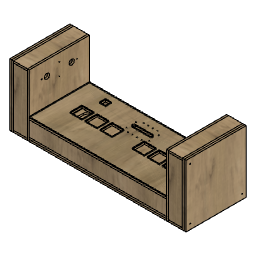
ongekicon-diy (Autodesk Fusion 360 design; units mm, degrees)
Autodesk Fusion 360 part; units mm, degrees
sketch "스케치1" plane through (0, 0, 0) normal (0, 0, 1) x (1, 0, 0)
  line L0 (289, -642.7336) -> (375, -642.7336)
  line L1 (375, -656.7336) -> (289, -656.7336)
  arc A0 (289, -642.7336) -> (289, -656.7336) centre (289, -649.7336) ccw
  arc A1 (375, -656.7336) -> (375, -642.7336) centre (375, -649.7336) ccw
  arc A2 (375, -656.7336) -> (375, -642.7336) centre (375, -649.7336) ccw
  circle A3 centre (277.0783, -626.5501) radius 2.65
  circle A4 centre (277.0783, -672.9171) radius 2.65
  circle A5 centre (386.9217, -626.4866) radius 2.65
  circle A6 centre (386.9217, -672.8535) radius 2.65
  circle A7 centre (299.0783, -611.6097) radius 2.65
  circle A8 centre (321.0783, -611.6097) radius 2.65
  circle A9 centre (343.0783, -611.6097) radius 2.65
  circle A10 centre (365.0783, -611.6097) radius 2.65
  circle A11 centre (364.9217, -687.7939) radius 2.65
  circle A12 centre (342.9217, -687.7939) radius 2.65
  circle A13 centre (320.9217, -687.7939) radius 2.65
  circle A14 centre (298.9217, -687.7939) radius 2.65
  line L2 (0, -575) -> (664, -575)
  line L3 (664, -575) -> (664, -866)
  line L4 (664, -866) -> (0, -866)
  line L5 (0, -866) -> (0, -575)
  line L6 (0, -1260) -> (664, -1260)
  line L7 (664, -1260) -> (664, -1333)
  line L8 (664, -1333) -> (0, -1333)
  line L9 (0, -1333) -> (0, -1260)
  line L10 (0, -1495) -> (0, -1422)
  line L11 (664, -1422) -> (664, -1495)
  line L12 (0, -1422) -> (664, -1422)
  line L13 (664, -1495) -> (0, -1495)
  line L14 (634, -431) -> (634, -260)
  line L15 (664, -200) -> (664, -491)
  line L16 (0, -200) -> (664, -200)
  line L17 (60, -461) -> (604, -461)
  line L18 (664, -491) -> (0, -491)
  line L19 (30, -260) -> (30, -431)
  line L20 (604, -230) -> (60, -230)
  line L21 (0, -491) -> (0, -200)
  line L22 (0, -230) -> (0, -200) construction
  arc A15 (60, -230) -> (30, -260) centre (60, -260) ccw
  arc A16 (634, -260) -> (604, -230) centre (604, -260) ccw
  arc A17 (604, -461) -> (634, -431) centre (604, -431) ccw
  arc A18 (30, -431) -> (60, -461) centre (60, -431) ccw
  circle A19 centre (644.0002, -219.9998) radius 3.25
  circle A20 centre (644.0002, -471.0002) radius 3.25
  circle A21 centre (19.9998, -219.9998) radius 3.25
  circle A22 centre (19.9998, -471.0002) radius 3.25
  line L23 (1115.742, -1032.7777) -> (1406.742, -1032.7777)
  line L24 (1406.742, -1032.7777) -> (1406.742, -1099.7777)
  line L25 (1406.742, -1099.7777) -> (1115.742, -1099.7777)
  line L26 (1115.742, -1099.7777) -> (1115.742, -1032.7777)
  line L27 (765.742, -1032.7777) -> (1056.742, -1032.7777)
  line L28 (1056.742, -1032.7777) -> (1056.742, -1099.7777)
  line L29 (1056.742, -1099.7777) -> (765.742, -1099.7777)
  line L30 (765.742, -1099.7777) -> (765.742, -1032.7777)
  line L31 (1115.742, -232.7777) -> (1406.742, -232.7777)
  line L32 (1406.742, -232.7777) -> (1406.742, -299.7777)
  line L33 (1406.742, -299.7777) -> (1115.742, -299.7777)
  line L34 (1115.742, -299.7777) -> (1115.742, -232.7777)
  line L35 (765.742, -232.7777) -> (1056.742, -232.7777)
  line L36 (1056.742, -232.7777) -> (1056.742, -299.7777)
  line L37 (1056.742, -299.7777) -> (765.742, -299.7777)
  line L38 (765.742, -299.7777) -> (765.742, -232.7777)
  line L39 (1455.3395, -732.946) -> (1522.3395, -732.946)
  line L40 (1522.3395, -732.946) -> (1522.3395, -1014.946)
  line L41 (1522.3395, -1014.946) -> (1455.3395, -1014.946)
  line L42 (1455.3395, -1014.946) -> (1455.3395, -732.946)
  line L43 (1622.3395, -1014.946) -> (1555.3395, -1014.946)
  line L44 (1555.3395, -1014.946) -> (1555.3395, -732.946)
  line L45 (1555.3395, -732.946) -> (1622.3395, -732.946)
  line L46 (1622.3395, -732.946) -> (1622.3395, -1014.946)
  line L47 (1555.3395, -664.946) -> (1555.3395, -382.946)
  line L48 (1555.3395, -382.946) -> (1622.3395, -382.946)
  line L49 (1622.3395, -382.946) -> (1622.3395, -664.946)
  line L50 (1622.3395, -664.946) -> (1555.3395, -664.946)
  line L51 (1455.3395, -664.946) -> (1455.3395, -382.946)
  line L52 (1455.3395, -382.946) -> (1522.3395, -382.946)
  line L53 (1522.3395, -664.946) -> (1455.3395, -664.946)
  line L54 (1522.3395, -382.946) -> (1522.3395, -664.946)
  line L55 (774.742, -665.946) -> (765.742, -665.946)
  line L56 (1047.742, -665.946) -> (774.742, -665.946)
  line L57 (1047.742, -665.946) -> (1056.742, -665.946)
  line L58 (1056.742, -365.946) -> (1056.742, -665.946)
  line L59 (1056.742, -365.946) -> (765.742, -365.946)
  line L60 (765.742, -365.946) -> (765.742, -665.946)
  arc A23 (1710.7461, -923.4722) -> (1740.7461, -953.4722) centre (1740.7461, -923.4722) ccw
  line L61 (1920.7461, -713.4722) -> (1740.7461, -713.4722)
  arc A24 (1740.7461, -713.4722) -> (1710.7461, -743.4722) centre (1740.7461, -743.4722) ccw
  line L62 (1710.7461, -743.4722) -> (1710.7461, -923.4722)
  circle A25 centre (1705.2461, -958.9722) radius 3.25
  circle A26 centre (1705.2461, -707.9722) radius 3.25
  line L63 (1685.2461, -683.4722) -> (1685.2461, -983.4722)
  line L64 (1976.2461, -683.4722) -> (1976.2461, -983.4722)
  line L65 (1950.7461, -923.4722) -> (1950.7461, -743.4722)
  line L66 (1740.7461, -953.4722) -> (1920.7461, -953.4722)
  arc A27 (1920.7461, -953.4722) -> (1950.7461, -923.4722) centre (1920.7461, -923.4722) ccw
  arc A28 (1950.7461, -743.4722) -> (1920.7461, -713.4722) centre (1920.7461, -743.4722) ccw
  circle A29 centre (1956.2461, -707.9722) radius 3.25
  circle A30 centre (1956.2461, -958.9722) radius 3.25
  line L67 (1976.2461, -683.4722) -> (1685.2461, -683.4722)
  line L68 (1976.2461, -983.4722) -> (1685.2461, -983.4722)
  line L69 (1976.2461, -633.4722) -> (1685.2461, -633.4722)
  line L70 (1976.2461, -333.4722) -> (1976.2461, -633.4722)
  line L71 (1710.7461, -393.4722) -> (1710.7461, -573.4722)
  line L72 (1685.2461, -333.4722) -> (1685.2461, -633.4722)
  arc A31 (1950.7461, -393.4722) -> (1920.7461, -363.4722) centre (1920.7461, -393.4722) ccw
  circle A32 centre (1956.2461, -608.9722) radius 3.25
  circle A33 centre (1705.2461, -357.9722) radius 3.25
  circle A34 centre (1956.2461, -357.9722) radius 3.25
  line L73 (1740.7461, -603.4722) -> (1920.7461, -603.4722)
  line L74 (1950.7461, -573.4722) -> (1950.7461, -393.4722)
  arc A35 (1920.7461, -603.4722) -> (1950.7461, -573.4722) centre (1920.7461, -573.4722) ccw
  line L75 (1920.7461, -363.4722) -> (1740.7461, -363.4722)
  circle A36 centre (1705.2461, -608.9722) radius 3.25
  arc A37 (1710.7461, -573.4722) -> (1740.7461, -603.4722) centre (1740.7461, -573.4722) ccw
  arc A38 (1740.7461, -363.4722) -> (1710.7461, -393.4722) centre (1740.7461, -393.4722) ccw
  line L76 (1976.2461, -333.4722) -> (1685.2461, -333.4722)
  line L77 (765.742, -704.946) -> (765.742, -1004.946)
  circle A39 centre (851.242, -774.446) radius 12.5
  line L78 (1056.742, -704.946) -> (765.742, -704.946)
  line L79 (1056.742, -1004.946) -> (765.742, -1004.946)
  circle A40 centre (971.242, -774.446) radius 12.5
  line L80 (765.742, -909.446) -> (765.742, -1004.946)
  circle A41 centre (996.242, -774.446) radius 2.2361
  circle A42 centre (826.242, -774.446) radius 2.2592
  circle A43 centre (911.242, -804.446) radius 2.2361
  line L81 (1056.742, -704.946) -> (1056.742, -1004.946)
  circle A44 centre (911.242, -744.446) radius 2.2361
  circle A45 centre (785.742, -641.446) radius 2.5
  circle A46 centre (1036.742, -641.446) radius 2.5
  circle A47 centre (1036.742, -390.446) radius 2.5
  circle A48 centre (1135.742, -390.446) radius 2.5
  line L82 (1115.742, -365.946) -> (1115.742, -665.946)
  circle A49 centre (1135.742, -641.446) radius 2.5
  line L83 (1397.742, -665.946) -> (1406.742, -665.946)
  line L84 (1397.742, -665.946) -> (1124.742, -665.946)
  line L85 (1406.742, -365.946) -> (1115.742, -365.946)
  line L86 (1406.742, -365.946) -> (1406.742, -665.946)
  line L87 (1124.742, -665.946) -> (1115.742, -665.946)
  circle A50 centre (1386.742, -641.446) radius 2.5
  circle A51 centre (1386.742, -390.446) radius 2.5
  circle A52 centre (456.3298, -1576.2079) radius 4
  circle A53 centre (547.3298, -1605.2079) radius 4
  circle A54 centre (592.8298, -1590.7079) radius 4
  circle A55 centre (547.3298, -1576.2079) radius 4
  circle A56 centre (410.8298, -1590.7079) radius 4
  circle A57 centre (501.8298, -1590.7079) radius 4
  circle A58 centre (456.3298, -1605.2079) radius 4
  line L88 (521.8298, -1571.2079) -> (481.2298, -1571.2079)
  line L89 (479.3298, -1573.1079) -> (479.3298, -1578.7079)
  line L90 (481.8298, -1581.2079) -> (521.8298, -1581.2079)
  line L91 (524.3298, -1578.7079) -> (524.3298, -1573.7079)
  arc A59 (524.3298, -1573.7079) -> (521.8298, -1571.2079) centre (521.8298, -1573.7079) ccw
  arc A60 (521.8298, -1581.2079) -> (524.3298, -1578.7079) centre (521.8298, -1578.7079) ccw
  arc A61 (479.3298, -1578.7079) -> (481.8298, -1581.2079) centre (481.8298, -1578.7079) ccw
  arc A62 (481.2298, -1571.2079) -> (479.3298, -1573.1079) centre (481.2298, -1573.1079) ccw
  line L92 (365.3298, -1554.2079) -> (638.3298, -1554.2079)
  line L93 (638.3298, -1554.2079) -> (638.3298, -1627.2079)
  line L94 (638.3298, -1627.2079) -> (365.3298, -1627.2079)
  line L95 (365.3298, -1627.2079) -> (365.3298, -1554.2079)
  arc A63 (933.742, -933.446) -> (931.242, -930.946) centre (931.242, -933.446) ccw
  line L96 (933.742, -938.446) -> (933.742, -933.446)
  line L97 (931.242, -930.946) -> (890.642, -930.946)
  arc A64 (931.242, -940.946) -> (933.742, -938.446) centre (931.242, -938.446) ccw
  arc A65 (888.742, -938.446) -> (891.242, -940.946) centre (891.242, -938.446) ccw
  circle A66 centre (865.742, -964.946) radius 4
  circle A67 centre (911.242, -950.446) radius 4
  line L98 (891.242, -940.946) -> (931.242, -940.946)
  arc A68 (890.642, -930.946) -> (888.742, -932.846) centre (890.642, -932.846) ccw
  circle A69 centre (865.742, -935.946) radius 4
  line L99 (888.742, -932.846) -> (888.742, -938.446)
  circle A70 centre (820.242, -950.446) radius 4
  circle A71 centre (1002.242, -950.446) radius 4
  circle A72 centre (956.742, -964.946) radius 4
  circle A73 centre (956.742, -935.946) radius 4
  circle A74 centre (1352.242, -950.446) radius 4
  circle A75 centre (1306.742, -935.946) radius 4
  arc A76 (1281.242, -940.946) -> (1283.742, -938.446) centre (1281.242, -938.446) ccw
  arc A77 (1283.742, -933.446) -> (1281.242, -930.946) centre (1281.242, -933.446) ccw
  line L100 (1281.242, -930.946) -> (1240.642, -930.946)
  circle A78 centre (1261.242, -950.446) radius 4
  circle A79 centre (1306.742, -964.946) radius 4
  line L101 (1406.742, -704.946) -> (1406.742, -1004.946)
  arc A80 (1238.742, -938.446) -> (1241.242, -940.946) centre (1241.242, -938.446) ccw
  circle A81 centre (1170.242, -950.446) radius 4
  line L102 (1283.742, -938.446) -> (1283.742, -933.446)
  circle A82 centre (1261.242, -744.446) radius 2.2361
  circle A83 centre (1215.742, -935.946) radius 4
  arc A84 (1240.642, -930.946) -> (1238.742, -932.846) centre (1240.642, -932.846) ccw
  line L103 (1238.742, -932.846) -> (1238.742, -938.446)
  circle A85 centre (1215.742, -964.946) radius 4
  circle A86 centre (1261.242, -804.446) radius 2.2361
  circle A87 centre (1176.242, -774.446) radius 2.2592
  line L104 (1241.242, -940.946) -> (1281.242, -940.946)
  circle A88 centre (1201.242, -774.446) radius 12.5
  line L105 (1406.742, -1004.946) -> (1115.742, -1004.946)
  line L106 (1115.742, -909.446) -> (1115.742, -1004.946)
  line L107 (1115.742, -704.946) -> (1115.742, -1004.946)
  line L108 (1406.742, -704.946) -> (1115.742, -704.946)
  circle A89 centre (1346.242, -774.446) radius 2.2361
  circle A90 centre (1321.242, -774.446) radius 12.5
  line L109 (121.8298, -1581.2079) -> (161.8298, -1581.2079)
  line L110 (161.8298, -1571.2079) -> (121.2298, -1571.2079)
  line L111 (119.3298, -1573.1079) -> (119.3298, -1578.7079)
  line L112 (278.3298, -1554.2079) -> (278.3298, -1627.2079)
  arc A91 (161.8298, -1581.2079) -> (164.3298, -1578.7079) centre (161.8298, -1578.7079) ccw
  arc A92 (119.3298, -1578.7079) -> (121.8298, -1581.2079) centre (121.8298, -1578.7079) ccw
  circle A93 centre (187.3298, -1576.2079) radius 4
  arc A94 (121.2298, -1571.2079) -> (119.3298, -1573.1079) centre (121.2298, -1573.1079) ccw
  line L113 (164.3298, -1578.7079) -> (164.3298, -1573.7079)
  circle A95 centre (187.3298, -1605.2079) radius 4
  circle A96 centre (141.8298, -1590.7079) radius 4
  arc A97 (164.3298, -1573.7079) -> (161.8298, -1571.2079) centre (161.8298, -1573.7079) ccw
  line L114 (278.3298, -1627.2079) -> (5.3298, -1627.2079)
  circle A98 centre (96.3298, -1576.2079) radius 4
  circle A99 centre (232.8298, -1590.7079) radius 4
  line L115 (5.3298, -1627.2079) -> (5.3298, -1554.2079)
  circle A100 centre (50.8298, -1590.7079) radius 4
  circle A101 centre (96.3298, -1605.2079) radius 4
  line L116 (5.3298, -1554.2079) -> (278.3298, -1554.2079)
  line L117 (138.1898, -635.6975) -> (109.1898, -635.6975)
  line L118 (109.1898, -635.6975) -> (109.1898, -606.6975)
  line L119 (109.1898, -606.6975) -> (138.1898, -606.6975)
  line L120 (138.1898, -606.6975) -> (138.1898, -635.6975)
  line L121 (525.8102, -635.6975) -> (554.8102, -635.6975)
  line L122 (554.8102, -635.6975) -> (554.8102, -606.6975)
  line L123 (554.8102, -606.6975) -> (525.8102, -606.6975)
  line L124 (525.8102, -606.6975) -> (525.8102, -635.6975)
  line L125 (554.8102, -985.6975) -> (554.8102, -956.6975)
  line L126 (109.1898, -985.6975) -> (109.1898, -956.6975)
  line L127 (138.1898, -956.6975) -> (138.1898, -985.6975)
  line L128 (525.8102, -956.6975) -> (525.8102, -985.6975)
  line L129 (525.8102, -985.6975) -> (554.8102, -985.6975)
  line L130 (664, -925) -> (664, -1216)
  line L131 (0, -1216) -> (0, -925)
  line L132 (109.1898, -956.6975) -> (138.1898, -956.6975)
  arc A102 (289, -992.7336) -> (289, -1006.7336) centre (289, -999.7336) ccw
  arc A103 (375, -1006.7336) -> (375, -992.7336) centre (375, -999.7336) ccw
  arc A104 (375, -1006.7336) -> (375, -992.7336) centre (375, -999.7336) ccw
  line L133 (138.1898, -985.6975) -> (109.1898, -985.6975)
  line L134 (375, -1006.7336) -> (289, -1006.7336)
  line L135 (664, -1216) -> (0, -1216)
  line L136 (0, -925) -> (664, -925)
  line L137 (289, -992.7336) -> (375, -992.7336)
  line L138 (554.8102, -956.6975) -> (525.8102, -956.6975)
  circle A105 centre (644, -130) radius 2.5
  circle A106 centre (644, 121) radius 2.5
  line L139 (664, 141) -> (664, -150)
  line L140 (0, 141) -> (664, 141)
  line L141 (664, -150) -> (0, -150)
  line L142 (0, -150) -> (0, 141)
  circle A107 centre (20, -130) radius 2.5
  circle A108 centre (20, 121) radius 2.5
  line L143 (180.5, -1312) -> (151.5, -1312)
  line L144 (151.5, -1312) -> (151.5, -1283)
  line L145 (151.5, -1283) -> (180.5, -1283)
  line L146 (180.5, -1283) -> (180.5, -1312)
  line L147 (318.75, -1303.75) -> (306.25, -1303.75)
  line L148 (306.25, -1303.75) -> (306.25, -1291.25)
  line L149 (306.25, -1291.25) -> (318.75, -1291.25)
  line L150 (318.75, -1291.25) -> (318.75, -1303.75)
  line L151 (483.5, -1312) -> (512.5, -1312)
  line L152 (512.5, -1312) -> (512.5, -1283)
  line L153 (483.5, -1283) -> (483.5, -1312)
  line L154 (512.5, -1283) -> (483.5, -1283)
  line L155 (357.75, -1303.75) -> (357.75, -1291.25)
  line L156 (357.75, -1291.25) -> (345.25, -1291.25)
  line L157 (345.25, -1303.75) -> (357.75, -1303.75)
  line L158 (345.25, -1291.25) -> (345.25, -1303.75)
  line L159 (136.915, -748.0793) -> (78.915, -748.0793)
  line L160 (78.915, -748.0793) -> (78.915, -690.0793)
  line L161 (78.915, -690.0793) -> (136.915, -690.0793)
  line L162 (136.915, -690.0793) -> (136.915, -748.0793)
  line L163 (209.8081, -748.0793) -> (151.8081, -748.0793)
  line L164 (151.8081, -748.0793) -> (151.8081, -690.0793)
  line L165 (151.8081, -690.0793) -> (209.8081, -690.0793)
  line L166 (209.8081, -690.0793) -> (209.8081, -748.0793)
  line L167 (282.7013, -748.0793) -> (224.7013, -748.0793)
  line L168 (224.7013, -748.0793) -> (224.7013, -690.0793)
  line L169 (224.7013, -690.0793) -> (282.7013, -690.0793)
  line L170 (282.7013, -690.0793) -> (282.7013, -748.0793)
  line L171 (512.1919, -690.0793) -> (454.1919, -690.0793)
  line L172 (527.085, -748.0793) -> (585.085, -748.0793)
  line L173 (454.1919, -748.0793) -> (512.1919, -748.0793)
  line L174 (585.085, -748.0793) -> (585.085, -690.0793)
  line L175 (381.2987, -690.0793) -> (381.2987, -748.0793)
  line L176 (381.2987, -748.0793) -> (439.2987, -748.0793)
  line L177 (454.1919, -690.0793) -> (454.1919, -748.0793)
  line L178 (585.085, -690.0793) -> (527.085, -690.0793)
  line L179 (439.2987, -690.0793) -> (381.2987, -690.0793)
  line L180 (527.085, -690.0793) -> (527.085, -748.0793)
  line L181 (512.1919, -748.0793) -> (512.1919, -690.0793)
  line L182 (439.2987, -748.0793) -> (439.2987, -690.0793)
  line L183 (152.5581, -1098.8293) -> (152.5581, -1040.8293)
  line L184 (79.665, -1098.8293) -> (79.665, -1040.8293)
  line L185 (79.665, -1040.8293) -> (137.665, -1040.8293)
  line L186 (152.5581, -1040.8293) -> (210.5581, -1040.8293)
  line L187 (137.665, -1040.8293) -> (137.665, -1098.8293)
  line L188 (210.5581, -1098.8293) -> (152.5581, -1098.8293)
  line L189 (137.665, -1098.8293) -> (79.665, -1098.8293)
  line L190 (210.5581, -1040.8293) -> (210.5581, -1098.8293)
  line L191 (225.4513, -1098.8293) -> (225.4513, -1040.8293)
  line L192 (283.4513, -1098.8293) -> (225.4513, -1098.8293)
  line L193 (225.4513, -1040.8293) -> (283.4513, -1040.8293)
  line L194 (283.4513, -1040.8293) -> (283.4513, -1098.8293)
  line L195 (526.335, -1098.8293) -> (584.335, -1098.8293)
  line L196 (526.335, -1040.8293) -> (526.335, -1098.8293)
  line L197 (380.5487, -1040.8293) -> (380.5487, -1098.8293)
  line L198 (380.5487, -1098.8293) -> (438.5487, -1098.8293)
  line L199 (453.4419, -1040.8293) -> (453.4419, -1098.8293)
  line L200 (438.5487, -1098.8293) -> (438.5487, -1040.8293)
  line L201 (438.5487, -1040.8293) -> (380.5487, -1040.8293)
  line L202 (511.4419, -1098.8293) -> (511.4419, -1040.8293)
  line L203 (453.4419, -1098.8293) -> (511.4419, -1098.8293)
  line L204 (584.335, -1098.8293) -> (584.335, -1040.8293)
  line L205 (511.4419, -1040.8293) -> (453.4419, -1040.8293)
  line L206 (584.335, -1040.8293) -> (526.335, -1040.8293)
  circle A109 centre (785.742, -390.446) radius 2.6
  line L207 (-100, 300) -> (2100, 300) construction
  line L208 (2100, 300) -> (2100, -1700) construction
  line L209 (2100, -1700) -> (-100, -1700) construction
  line L210 (-100, -1700) -> (-100, 300) construction
  line L211 (725, -150) -> (2000, -150) construction
  line L212 (2000, -150) -> (2000, -1125) construction
  line L213 (2000, -1125) -> (725, -1125) construction
  line L214 (725, -1125) -> (725, -150) construction
  line L215 (668.8847, -1871.4967) -> (1168.8847, -1871.4967) construction
  line L216 (1168.8847, -1871.4967) -> (1168.8847, -1771.4967) construction
  line L217 (1168.8847, -1771.4967) -> (668.8847, -1771.4967) construction
  line L218 (668.8847, -1771.4967) -> (668.8847, -1871.4967) construction
  line L219 (150.0308, -1682.8385) -> (548.5377, -1682.465) construction
  line L220 (548.5377, -1682.465) -> (548.5069, -1649.6265) construction
  line L221 (548.5069, -1649.6265) -> (150, -1650) construction
  line L222 (150, -1650) -> (150.0308, -1682.8385) construction
  line L223 (918.4716, -1223.3511) -> (1893.2087, -1220.0773) construction
  line L224 (1893.2087, -1220.0773) -> (1892.9571, -1145.174) construction
  line L225 (1892.9571, -1145.174) -> (918.22, -1148.4477) construction
  line L226 (918.22, -1148.4477) -> (918.4716, -1223.3511) construction
  point P0 (0, -350)
  point P1 (1830.7461, -483.4722)
  point P2 (911.242, -951.946)
  point P3 (911.242, -951.946)
  point P4 (166, -1297.5)
  point P5 (166, -1297.5)
  point P6 (501.8298, -1590.7079)
  point P7 (501.8298, -1576.2079)
  point P8 (911.242, -935.946)
  point P9 (911.242, -950.446)
  point P10 (1261.242, -951.946)
  point P11 (1261.242, -935.946)
  point P12 (1261.242, -950.446)
  point P13 (1261.242, -951.946)
  point P14 (141.8298, -1576.2079)
  point P15 (141.8298, -1590.7079)
  point P16 (540.3102, -621.1975)
  point P17 (253.7013, -719.0793)
  point P18 (107.915, -719.0793)
  point P19 (123.6898, -621.1975)
  point P20 (107.915, -719.0793)
  point P21 (253.7013, -719.0793)
  point P22 (123.6898, -621.1975)
  point P23 (540.3102, -621.1975)
  point P24 (123.6898, -621.1975)
  point P25 (540.3102, -621.1975)
  point P26 (166, -1297.5)
  point P27 (107.915, -719.0793)
  point P28 (180.8081, -719.0793)
  point P29 (253.7013, -719.0793)
  point P30 (556.085, -719.0793)
  point P31 (410.2987, -719.0793)
  point P32 (556.085, -719.0793)
  point P33 (410.2987, -719.0793)
  point P34 (410.2987, -719.0793)
  point P35 (483.1919, -719.0793)
  point P36 (556.085, -719.0793)
  point P37 (79.665, -1040.8293)
  dimension "d11" = 7
  dimension "d22" = 5.3
  dimension "d23" = 5.3
  dimension "d24" = 5.3
  dimension "d25" = 5.3
  dimension "d26" = 5.3
  dimension "d27" = 22
  dimension "d28" = 22
  dimension "d29" = 22
  dimension "d33" = 5.3
  dimension "d34" = 5.3
  dimension "d35" = 5.3
  dimension "d36" = 5.3
  dimension "d37" = 5.3
  dimension "d38" = 5.3
  dimension "d39" = 5.3
  dimension "d43" = 291
  dimension "d64" = 86
  dimension "d194" = 73
  dimension "d195" = 664
  dimension "d196" = 73
  dimension "d362" = 291
  dimension "d364" = 28.284
  dimension "d365" = 28.284
  dimension "d366" = 28.284
  dimension "d367" = 28.284
  dimension "d372" = 30
  dimension "d373" = 30
  dimension "d374" = 30
  dimension "d375" = 30
  dimension "d376" = 6.5
  dimension "d377" = 6.5
  dimension "d382" = 6.5
  dimension "d383" = 6.5
  dimension "d537" = 664
  dimension "d553" = 67
  dimension "d554" = 67
  dimension "d555" = 67
  dimension "d556" = 67
  dimension "d807" = 300
  dimension "d858" = 30
  dimension "d859" = 30
  dimension "d860" = 30
  dimension "d861" = 30
  dimension "d862" = 6.5
  dimension "d863" = 6.5
  dimension "d865" = 6.5
  dimension "d884" = 6.5
  dimension "d892" = 30
  dimension "d893" = 30
  dimension "d894" = 30
  dimension "d895" = 30
  dimension "d896" = 6.5
  dimension "d897" = 6.5
  dimension "d898" = 6.5
  dimension "d907" = 6.5
  dimension "d943" = 25
  dimension "d944" = 25
  dimension "d954" = 5
  dimension "d955" = 5
  dimension "d956" = 5
  dimension "d957" = 300
  dimension "d966" = 5
  dimension "d967" = 5
  dimension "d968" = 5
  dimension "d969" = 5
  dimension "d1011" = 8
  dimension "d1012" = 8
  dimension "d1013" = 8
  dimension "d1014" = 8
  dimension "d1015" = 8
  dimension "d1016" = 8
  dimension "d1017" = 8
  dimension "d1055" = 2.5
  dimension "d1056" = 1.9
  dimension "d1057" = 273
  dimension "d1058" = 73
  dimension "d1059" = 8
  dimension "d1060" = 8
  dimension "d1061" = 8
  dimension "d1062" = 8
  dimension "d1063" = 8
  dimension "d1064" = 8
  dimension "d1065" = 8
  dimension "d1072" = 2.5
  dimension "d1073" = 1.9
  dimension "d1094" = 25
  dimension "d1095" = 25
  dimension "d1096" = 8
  dimension "d1097" = 8
  dimension "d1098" = 8
  dimension "d1099" = 8
  dimension "d1100" = 8
  dimension "d1101" = 8
  dimension "d1102" = 8
  dimension "d1105" = 2.5
  dimension "d1106" = 1.9
  dimension "d1111" = 8
  dimension "d1112" = 8
  dimension "d1113" = 8
  dimension "d1114" = 8
  dimension "d1115" = 8
  dimension "d1116" = 8
  dimension "d1117" = 8
  dimension "d1124" = 2.5
  dimension "d1125" = 1.9
  dimension "d1126" = 273
  dimension "d1127" = 73
  dimension "d1144" = 29
  dimension "d1145" = 29
  dimension "d1146" = 29
  dimension "d1147" = 29
  dimension "d1148" = 7
  dimension "d1171" = 291
  dimension "d1197" = 664
  dimension "d1210" = 29
  dimension "d1211" = 29
  dimension "d1212" = 29
  dimension "d1213" = 29
  dimension "d1237" = 291
  dimension "d1259" = 5
  dimension "d1260" = 5
  dimension "d1261" = 5
  dimension "d1262" = 5
  dimension "d1263" = 664
  dimension "d1322" = 29
  dimension "d1323" = 29
  dimension "d1324" = 12.5
  dimension "d1325" = 12.5
  dimension "d1326" = 58
  dimension "d1327" = 58
  dimension "d1328" = 58
  dimension "d1329" = 58
  dimension "d1330" = 58
  dimension "d1331" = 58
  dimension "d1335" = 58
  dimension "d1336" = 58
  dimension "d1337" = 58
  dimension "d1338" = 58
  dimension "d1339" = 58
  dimension "d1340" = 58
  dimension "d1347" = 5.2
  dimension "d1348" = 100
  dimension "d1349" = 50
  dimension "d1350" = 50
  constraint horizontal L0
  constraint horizontal L1
  constraint tangent L0 A0
  constraint tangent L1 A0
  constraint tangent L0 A1
  constraint tangent L1 A1
  constraint horizontal L2
  constraint vertical L3
  constraint horizontal L4
  constraint vertical L5
  constraint horizontal L6
  constraint vertical L7
  constraint horizontal L8
  constraint vertical L9
  constraint horizontal L12
  constraint vertical L11
  constraint horizontal L13
  constraint vertical L10
  constraint horizontal L16
  constraint vertical L15
  constraint horizontal L18
  constraint vertical L21
  constraint horizontal L20
  constraint perpendicular L19 L20
  constraint parallel L17 L20
  constraint parallel L14 L19
  constraint vertical L22
  constraint tangent L20 A15
  constraint tangent L19 A15
  constraint tangent L20 A16
  constraint tangent L14 A16
  constraint tangent L14 A17
  constraint tangent L17 A17
  constraint tangent L19 A18
  constraint tangent L17 A18
  constraint horizontal L23
  constraint vertical L24
  constraint horizontal L25
  constraint vertical L26
  constraint horizontal L27
  constraint vertical L28
  constraint horizontal L29
  constraint vertical L30
  constraint horizontal L31
  constraint vertical L32
  constraint horizontal L33
  constraint vertical L34
  constraint horizontal L35
  constraint vertical L36
  constraint horizontal L37
  constraint vertical L38
  constraint horizontal L39
  constraint vertical L40
  constraint horizontal L41
  constraint vertical L42
  constraint horizontal L45
  constraint vertical L46
  constraint horizontal L43
  constraint vertical L44
  constraint horizontal L52
  constraint vertical L54
  constraint horizontal L53
  constraint vertical L51
  constraint horizontal L48
  constraint vertical L49
  constraint horizontal L50
  constraint vertical L47
  constraint vertical L60
  constraint vertical L58
  constraint horizontal L56
  constraint perpendicular L57 L58
  constraint perpendicular L55 L60
  constraint horizontal L59
  constraint vertical L63
  constraint vertical L64
  constraint horizontal L61
  constraint perpendicular L61 L62
  constraint parallel L61 L66
  constraint parallel L62 L65
  constraint tangent L61 A24
  constraint tangent A24 L62
  constraint tangent L61 A28
  constraint tangent L65 A28
  constraint tangent A23 L62
  constraint tangent A23 L66
  constraint tangent L65 A27
  constraint tangent L66 A27
  constraint horizontal L67
  constraint horizontal L68
  constraint vertical L72
  constraint vertical L70
  constraint horizontal L75
  constraint perpendicular L71 L75
  constraint parallel L73 L75
  constraint parallel L71 L74
  constraint tangent L75 A38
  constraint tangent L71 A38
  constraint tangent A31 L75
  constraint tangent A31 L74
  constraint tangent L71 A37
  constraint tangent L73 A37
  constraint tangent L74 A35
  constraint tangent L73 A35
  constraint horizontal L76
  constraint horizontal L69
  constraint vertical L77
  constraint vertical L81
  constraint vertical L80
  constraint horizontal L78
  constraint horizontal L79
  constraint vertical L82
  constraint vertical L86
  constraint horizontal L84
  constraint perpendicular L83 L86
  constraint perpendicular L82 L87
  constraint horizontal L85
  constraint coincident P26 P5
  constraint coincident P6 A57.centre
  constraint horizontal L88
  constraint perpendicular L88 L89
  constraint parallel L88 L90
  constraint parallel L89 L91
  constraint tangent L91 A59
  constraint tangent L88 A59
  constraint tangent L91 A60
  constraint tangent L90 A60
  constraint equal A59 A60
  constraint tangent L89 A61
  constraint tangent L90 A61
  constraint equal A59 A61
  constraint tangent L88 A62
  constraint tangent L89 A62
  constraint horizontal L92
  constraint vertical L93
  constraint horizontal L94
  constraint vertical L95
  constraint coincident P9 A67.centre
  constraint horizontal L97
  constraint perpendicular L97 L99
  constraint parallel L97 L98
  constraint parallel L96 L99
  constraint tangent A63 L96
  constraint tangent A63 L97
  constraint tangent L96 A64
  constraint tangent A64 L98
  constraint equal A63 A64
  constraint tangent A65 L99
  constraint tangent A65 L98
  constraint equal A63 A65
  constraint tangent L97 A68
  constraint tangent A68 L99
  constraint vertical L107
  constraint vertical L101
  constraint vertical L106
  constraint horizontal L108
  constraint horizontal L105
  constraint coincident P12 A78.centre
  constraint horizontal L100
  constraint perpendicular L100 L103
  constraint parallel L100 L104
  constraint parallel L102 L103
  constraint tangent A77 L102
  constraint tangent A77 L100
  constraint tangent A76 L102
  constraint tangent A76 L104
  constraint equal A76 A77
  constraint tangent A80 L103
  constraint tangent A80 L104
  constraint equal A77 A80
  constraint tangent L100 A84
  constraint tangent A84 L103
  constraint coincident P15 A96.centre
  constraint horizontal L110
  constraint perpendicular L110 L111
  constraint parallel L109 L110
  constraint parallel L111 L113
  constraint tangent L113 A97
  constraint tangent L110 A97
  constraint tangent A91 L113
  constraint tangent L109 A91
  constraint equal A91 A97
  constraint tangent L111 A92
  constraint tangent L109 A92
  constraint equal A92 A97
  constraint tangent L110 A94
  constraint tangent L111 A94
  constraint horizontal L116
  constraint vertical L112
  constraint horizontal L114
  constraint vertical L115
  constraint coincident P27 P20
  constraint coincident P29 P21
  constraint coincident P24 P22
  constraint coincident P25 P23
  constraint horizontal L117
  constraint perpendicular L117 L118
  constraint parallel L117 L119
  constraint parallel L118 L120
  constraint horizontal L121
  constraint perpendicular L121 L122
  constraint parallel L121 L123
  constraint parallel L122 L124
  constraint horizontal L137
  constraint horizontal L134
  constraint tangent A102 L137
  constraint tangent A102 L134
  constraint tangent A103 L137
  constraint tangent A103 L134
  constraint horizontal L136
  constraint vertical L130
  constraint horizontal L135
  constraint vertical L131
  constraint horizontal L133
  constraint perpendicular L126 L133
  constraint parallel L132 L133
  constraint parallel L126 L127
  constraint horizontal L129
  constraint perpendicular L125 L129
  constraint parallel L129 L138
  constraint parallel L125 L128
  constraint vertical L139
  constraint horizontal L141
  constraint vertical L142
  constraint horizontal L143
  constraint perpendicular L143 L144
  constraint parallel L143 L145
  constraint parallel L144 L146
  constraint horizontal L147
  constraint perpendicular L147 L148
  constraint parallel L147 L149
  constraint parallel L148 L150
  constraint horizontal L159
  constraint perpendicular L159 L160
  constraint parallel L159 L161
  constraint parallel L160 L162
  constraint horizontal L163
  constraint perpendicular L163 L164
  constraint parallel L163 L165
  constraint parallel L164 L166
  constraint horizontal L167
  constraint perpendicular L167 L168
  constraint parallel L167 L169
  constraint parallel L168 L170
  constraint horizontal L189
  constraint perpendicular L184 L189
  constraint parallel L185 L189
  constraint parallel L184 L187
  constraint horizontal L188
  constraint perpendicular L183 L188
  constraint parallel L186 L188
  constraint parallel L183 L190
  constraint horizontal L192
  constraint perpendicular L191 L192
  constraint parallel L192 L193
  constraint parallel L191 L194
  constraint coincident P37 L184.end
  constraint horizontal L207
  constraint vertical L208
  constraint horizontal L209
  constraint vertical L210
  constraint horizontal L211
  constraint vertical L212
  constraint horizontal L213
  constraint vertical L214
  measures "d11" radius of A0
  measures "d22" diameter of A3
  measures "d23" diameter of A4
  measures "d24" diameter of A5
  measures "d25" diameter of A6
  measures "d26" diameter of A7
  measures "d27" distance of A7.centre A8.centre
  measures "d28" distance of A8.centre A9.centre
  measures "d29" distance of A9.centre A10.centre
  measures "d33" diameter of A8
  measures "d34" diameter of A9
  measures "d35" diameter of A10
  measures "d36" diameter of A11
  measures "d37" diameter of A12
  measures "d38" diameter of A13
  measures "d39" diameter of A14
  measures "d43" distance of L2.start L4.end
  measures "d64" distance of A0.centre A1.centre
  measures "d194" distance of L6.start L8.end
  measures "d195" distance of L11.start L10.end
  measures "d196" distance of L10.start L10.end
  measures "d362" distance of L16.start L18.end
  measures "d364" distance of L15.end A20.centre
  measures "d365" distance of L15.start A19.centre
  measures "d366" distance of L16.start A21.centre
  measures "d367" distance of L18.end A22.centre
  measures "d372" radius of A15
  measures "d373" radius of A16
  measures "d374" radius of A17
  measures "d375" radius of A18
  measures "d376" diameter of A19
  measures "d377" diameter of A20
  measures "d382" diameter of A21
  measures "d383" diameter of A22
  measures "d537" distance of L2.start L2.end
  measures "d553" distance of L23.start L25.end
  measures "d554" distance of L27.start L29.end
  measures "d555" distance of L31.start L33.end
  measures "d556" distance of L35.start L37.end
  measures "d807" distance of L57.end L58.start
  measures "d858" radius of A24
  measures "d859" radius of A28
  measures "d860" radius of A23
  measures "d861" radius of A27
  measures "d862" diameter of A26
  measures "d863" diameter of A29
  measures "d865" diameter of A25
  measures "d884" diameter of A30
  measures "d892" radius of A38
  measures "d893" radius of A31
  measures "d894" radius of A37
  measures "d895" radius of A35
  measures "d896" diameter of A33
  measures "d897" diameter of A34
  measures "d898" diameter of A36
  measures "d907" diameter of A32
  measures "d943" diameter of A39
  measures "d944" diameter of A40
  measures "d954" diameter of A45
  measures "d955" diameter of A46
  measures "d956" diameter of A47
  measures "d957" distance of L85.start L83.end
  measures "d966" diameter of A48
  measures "d967" diameter of A49
  measures "d968" diameter of A50
  measures "d969" diameter of A51
  measures "d1011" diameter of A52
  measures "d1012" diameter of A58
  measures "d1013" diameter of A55
  measures "d1014" diameter of A53
  measures "d1015" diameter of A57
  measures "d1016" diameter of A56
  measures "d1017" diameter of A54
  measures "d1055" radius of A59
  measures "d1056" radius of A62
  measures "d1057" distance of L92.start L92.end
  measures "d1058" distance of L92.start L94.end
  measures "d1059" diameter of A69
  measures "d1060" diameter of A66
  measures "d1061" diameter of A73
  measures "d1062" diameter of A72
  measures "d1063" diameter of A67
  measures "d1064" diameter of A70
  measures "d1065" diameter of A71
  measures "d1072" radius of A63
  measures "d1073" radius of A68
  measures "d1094" diameter of A88
  measures "d1095" diameter of A90
  measures "d1096" diameter of A83
  measures "d1097" diameter of A85
  measures "d1098" diameter of A75
  measures "d1099" diameter of A79
  measures "d1100" diameter of A78
  measures "d1101" diameter of A81
  measures "d1102" diameter of A74
  measures "d1105" radius of A77
  measures "d1106" radius of A84
  measures "d1111" diameter of A98
  measures "d1112" diameter of A101
  measures "d1113" diameter of A93
  measures "d1114" diameter of A95
  measures "d1115" diameter of A96
  measures "d1116" diameter of A100
  measures "d1117" diameter of A99
  measures "d1124" radius of A97
  measures "d1125" radius of A94
  measures "d1126" distance of L115.end L112.start
  measures "d1127" distance of L115.end L114.end
  measures "d1144" distance of L118.end L119.end
  measures "d1145" distance of L117.end L118.end
  measures "d1146" distance of L122.end L123.end
  measures "d1147" distance of L121.end L122.end
  measures "d1148" radius of A102
  measures "d1171" distance of L131.start L131.end
  measures "d1197" distance of L130.start L131.end
  measures "d1210" distance of L126.end L127.start
  measures "d1211" distance of L126.end L126.start
  measures "d1212" distance of L128.start L125.end
  measures "d1213" distance of L125.start L125.end
  measures "d1237" distance of L141.end L140.start
  measures "d1259" diameter of A108
  measures "d1260" diameter of A106
  measures "d1261" diameter of A107
  measures "d1262" diameter of A105
  measures "d1263" distance of L139.start L140.start
  measures "d1322" distance of L144.end L145.end
  measures "d1323" distance of L143.end L144.end
  measures "d1324" distance of L148.end L149.end
  measures "d1325" distance of L147.end L148.end
  measures "d1326" distance of L160.end L161.end
  measures "d1327" distance of L159.end L160.end
  measures "d1328" distance of L164.end L165.end
  measures "d1329" distance of L163.end L164.end
  measures "d1330" distance of L168.end L169.end
  measures "d1331" distance of L167.end L168.end
  measures "d1335" distance of P37 L185.end
  measures "d1336" distance of P37 L184.start
  measures "d1337" distance of L186.end L183.end
  measures "d1338" distance of L183.start L183.end
  measures "d1339" distance of L193.end L191.end
  measures "d1340" distance of L191.start L191.end
  measures "d1347" diameter of A109
extrude "돌출62" add sketch "스케치1" along normal blind 5 contours L130 L131 L135 L136 makes body 1
extrude "돌출63" add sketch "스케치1" along normal blind 9 separate body contours L2 L3 L4 L5 | L6 L7 L8 L9 | L10 L11 L12 L13 | L15 L16 L18 L21 | L23 L24 L25 L26 | L27 L28 L29 L30 | L31 L32 L33 L34 | L35 L36 L37 L38 | L39 L40 L41 L42 | L43 L44 L45 L46 | L47 L48 L49 L50 | L51 L52 L53 L54 | L55 L56 L57 L58 L59 L60 | L63 L64 L67 L68 | L69 L70 L72 L76 | L77 L78 L79 L80 L81 | L82 L83 L84 L85 L86 L87 | L92 L93 L94 L95 | L101 L105 L106 L107 L108 | L112 L114 L115 L116 | L139 L140 L141 L142 | A109 makes body 2 at (1577.6728, -570.946, 0) makes body 3 at (862.742, -277.4444, 0) makes body 4 at (1389.6697, -886.0176, 0) makes body 5 at (624.4965, -1590.7079, 0) makes body 6 at (435.1019, -45.8828, 0) makes body 7 at (241.3333, -481, 0) makes body 8 at (264.4965, -1590.7079, 0) makes body 9 at (1220.1595, -474.7257, 0) makes body 10 at (1212.742, -277.4444, 0) makes body 11 at (1577.6728, -920.946, 0) makes body 12 at (1860.7461, -623.4722, 0) makes body 13 at (1477.6728, -570.946, 0) makes body 14 at (862.742, -1077.4444, 0) makes body 15 at (1039.6697, -886.0176, 0) makes body 16 at (50.5, -1292, 0) makes body 17 at (348.4329, -826.6931, 0) makes body 18 at (221.3333, -1446.3333, 0) makes body 19 at (862.4649, -465.645, 0) makes body 20 at (1212.742, -1077.4444, 0) makes body 21 at (1477.6728, -920.946, 0) makes body 22 at (1800.7461, -693.4722, 0)
move_body "정렬110" bodies 7 to x (1, 0, 0) y (0, 1, 0) z (0, 0, 1) at (0, 341, 9)
move_body "이동82" bodies 16 8 5 18 to x (1, 0, 0) y (0, 0, 1) z (0, -1, 0) at (0, -1213.5, 1218.5)
move_body "이동83" bodies 5 8 to x (0, -1, 0) y (1, 0, 0) z (0, 0, 1) at (1446.3298, -980.6702, 0)
move_body "정렬111" bodies 5 to x (1, 0, 0) y (0, 1, 0) z (0, 0, 1) at (431.1702, 1478, 426.7079)
move_body "정렬112" bodies 8 to x (1, 0, 0) y (0, 1, 0) z (0, 0, 1) at (-223.8298, 1118, 426.7079)
move_body "정렬113" bodies 16 to x (1, 0, 0) y (0, 1, 0) z (0, 0, 1) at (0, 1354.5, 132.5)
move_body "정렬114" bodies 18 to x (1, 0, 0) y (0, 1, 0) z (0, 0, 1) at (0, 1072.5, 294.5)
move_body "정렬115" bodies 17 to x (1, 0, 0) y (0, 1, 0) z (0, 0, 1) at (0, 716, 91)
move_body "정렬116" bodies 1 to x (1, 0, 0) y (0, 1, 0) z (0, 0, 1) at (0, 1066, 100)
move_body "이동84" bodies 3 10 12 20 22 9 4 19 15 14 to x (0, -1, 0) y (1, 0, 0) z (0, 0, 1) at (1628.7615, -195.7679, 0)
move_body "이동85" bodies 12 15 19 4 9 22 to x (0, 0, 1) y (0, 1, 0) z (-1, 0, 0) at (630.3286, 0, -630.3286)
move_body "정렬117" bodies 22 to x (1, 0, 0) y (0, 1, 0) z (0, 0, 1) at (-9, 569.5041, 317.5262)
move_body "정렬118" bodies 10 to x (1, 0, 0) y (0, 1, 0) z (0, 0, 1) at (-783.6553, 0, 332.487)
move_body "정렬119" bodies 4 to x (1, 0, 0) y (0, 1, 0) z (0, 0, 1) at (-85, 0, 339)
move_body "정렬120" bodies 15 to x (1, 0, 0) y (0, 1, 0) z (0, 0, 1) at (42.6714, 1102.5099, 6.513)
move_body "정렬121" bodies 14 to x (1, 0, 0) y (0, 1, 0) z (0, 0, 1) at (144.0162, 1102.5099, 0)
move_body "정렬122" bodies 12 to x (1, 0, 0) y (0, 1, 0) z (0, 0, 1) at (118.6714, 2022.014, -364.9608)
move_body "정렬123" bodies 19 to x (1, 0, 0) y (0, 1, 0) z (0, 0, 1) at (127.6714, 1102.5099, -332.487)
move_body "정렬124" bodies 20 to x (1, 0, 0) y (0, 1, 0) z (0, 0, 1) at (144.0162, 1452.5099, 291)
move_body "정렬125" bodies 4 to x (1, 0, 0) y (0, 1, 0) z (0, 0, 1) at (-545.3286, 1452.5099, -332.487)
move_body "정렬126" bodies 10 to x (1, 0, 0) y (0, 1, 0) z (0, 0, 1) at (-621.3286, 1452.5099, -332.487)
move_body "정렬127" bodies 22 to x (1, 0, 0) y (0, 1, 0) z (0, 0, 1) at (-697.3286, 1452.5099, -332.487)
move_body "정렬128" bodies 9 to x (1, 0, 0) y (0, 1, 0) z (0, 0, 1) at (-715.3286, 1452.5099, -332.487)
move_body "정렬129" bodies 3 to x (1, 0, 0) y (0, 1, 0) z (0, 0, 1) at (-1404.9838, 1102.5099, 291)
move_body "이동86" bodies 11 13 21 2 to x (1, 0, 0) y (0, 0, 1) z (0, -1, 0) at (0, -1481.933, 1490.933)
move_body "정렬130" bodies 21 to x (1, 0, 0) y (0, 1, 0) z (0, 0, 1) at (-782.3395, 1340.933, -466.987)
move_body "정렬131" bodies 11 to x (1, 0, 0) y (0, 1, 0) z (0, 0, 1) at (-882.3395, 1622.933, -466.987)
move_body "정렬132" bodies 2 to x (1, 0, 0) y (0, 1, 0) z (0, 0, 1) at (-1631.3395, 1622.933, -816.987)
move_body "정렬133" bodies 13 to x (1, 0, 0) y (0, 1, 0) z (0, 0, 1) at (-1531.3395, 1340.933, -816.987)
